Autodesk Fusion 360 part; units mm, degrees
(part 6 of 6)
  circle A1468 centre (-50.0063, 76.2) radius 1.1
  circle A1469 centre (30.9563, 76.2) radius 1.1
  circle A1470 centre (128.5875, 76.2) radius 1.1
  circle A1471 centre (128.5875, 14.2875) radius 1.1
  circle A1472 centre (107.1563, -26.1938) radius 1.1
  circle A1473 centre (26.1938, -26.1938) radius 1.1
  circle A1474 centre (-54.7687, -26.1938) radius 1.1
  circle A1475 centre (-178.5916, -47.625) radius 2.4872
  circle A1476 centre (-176.2125, -14.2875) radius 3.6059
  line L738 (-145, -39.5) -> (-166.8472, -39.5)
  line L739 (-166.8472, -39.5) -> (-166.8472, -28.5006)
  line L740 (-166.8472, -28.5006) -> (-145, -28.5006)
  line L741 (-145, -28.5006) -> (-145, -39.5)
extrude "Extrude2" cut sketch "sketch 18250" along normal blind 10 contours A0 A1470 | A88 A1469 | A186 A1471 | A324 A1468 | A452 A1467 | A616 A1466 | A652 A1465 | A931 A1472 | A979 A1458 | A981 A1459 | A1006 A1473 | A1054 A1460 | A1280 A1464 | A1287 A1476 | A1305 A1474 | A1353 A1461 | A1413 A1462 | A1457 A1463 | A1475 | L738 L739 L740 L741 picked at (-178.8533, -13.7545) bodies 1 makes body 2 at (314.5316, -44.135, 0.5) makes body 3 at (318.287, -10.2067, 0.5) makes body 4 at (315.747, -10.2067, 0.5)
